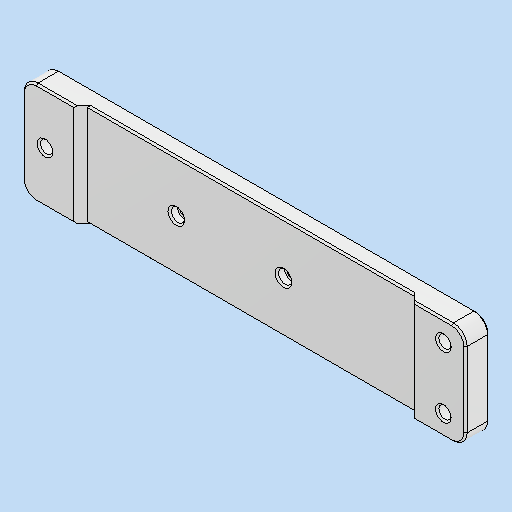
# Autodesk Inventor part: LRS-150-din-bracket
Saved by Autodesk Inventor 2026 (Build 300175050, 175E)
## iProperties
Created: 2025-06-13
Part Number: LRS-150-din-bracket
Material: ABS Plastic
Document SubType Name: Modeling
Designer: kuzmin
Density: 1.06 g/cm^3
Appearance: Smooth - White
Author: kuzmin
Autodesk Inventor part; units mm, degrees
ref_plane "YZ Plane" through (0, 0, 0) normal (1, 0, 0) x (0, 1, 0)
ref_plane "XZ Plane" through (0, 0, 0) normal (0, 1, 0) x (-1, 0, 0)
ref_plane "XY Plane" through (0, 0, 0) normal (0, 0, 1) x (1, 0, 0)
sketch "Sketch1" plane through (0, 0, 0) normal (0, 0, 1) x (1, 0, 0)
  line L0 (-65, 15) -> (65, 15)
  line L1 (65, 15) -> (65, -15)
  line L2 (65, -15) -> (-65, -15)
  line L3 (-65, -15) -> (-65, 15)
  point P0 (0, 0)
  point P1 (0, 15)
  point P2 (65, 0)
  dimension "d0" = 130
  dimension "d1" = 30
  constraints: 8 end point, 2 midpoint, 2 parallel, 1 horizontal, 1 horizontal alignment, 1 perpendicular, 1 vertical alignment
  measures "d0" distance of L0.start L0.end
  measures "d1" distance of L0.end L1.end
extrude "Extrusion1" add sketch "Sketch1" along normal blind 7
sketch "Sketch2" plane through (0, 0, 7) normal (0, 0, 1) x (1, 0, 0)
  line L0 (58.5, 9) -> (58.5, -9) construction
  line L1 (-58.5, 0) -> (58.5, 0) construction
  point P0 (0, 0)
  point P1 (0, 0)
  dimension "d4" = 117
  dimension "d5" = 18
  constraints: 4 coincident, 4 end point, 2 midpoint, 1 horizontal, 1 vertical
  measures "d4" distance of L1.start L1.end
  measures "d5" distance of L0.start L0.end
hole "Hole1" at (-58.5, 0, 7) at (58.5, 9, 7) at (58.5, -9, 7) direction (0, 0, -1) diameter 3.6 end through all
sketch "Sketch3" plane through (0, 0, 7) normal (0, 0, 1) x (1, 0, 0)
  line L0 (65, 15) -> (-65, 15) projected
  line L1 (-65, -15) -> (65, -15) projected
  line L2 (-50, 15) -> (50, 15)
  line L3 (50, 15) -> (50, -15)
  line L4 (50, -15) -> (-50, -15)
  line L5 (-50, -15) -> (-50, 15)
  point P0 (0, 0)
  point P1 (0, -15)
  dimension "d13" = 100
  constraints: 8 end point, 2 parallel, 2 point on line, 1 horizontal, 1 midpoint, 1 perpendicular, 1 vertical alignment
  measures "d13" distance between parallel lines of L3 L5
extrude "Extrusion2" cut sketch "Sketch3" against normal blind 2
sketch "Sketch4" plane through (0, 0, 5) normal (0, 0, 1) x (1, 0, 0)
  line L0 (-21.9201, 0) -> (9.5799, 0) construction
  point P0 (0, 0)
  dimension "d16" = 31.5
  constraints: 2 coincident, 2 end point, 1 horizontal
  measures "d16" distance of L0.start L0.end
hole "Hole2" at (-21.9201, 0, 5) at (9.5799, 0, 5) direction (0, 0, -1) diameter 2.5 end through all counterbore diameter 3.9 counterbore depth 2.3
fillet "Fillet1" radius 4 4 edges at (-65, -15, 3.5) (-65, 15, 3.5) (65, 15, 3.5) (65, -15, 3.5)
chamfer "Chamfer1" distance 2 angle 45 2 edges at (-50, 0, 5) (50, 0, 5)
chamfer "Chamfer2" distance 0.5 angle 45 10 edges at (-21.9201, 1.95, 5) (9.5799, 1.95, 5) (58.5, -7.2, 7) (58.5, 10.8, 7) (-58.5, 1.8, 7) (58.5, -7.2, 0) (-58.5, 1.8, 0) (58.5, 10.8, 0) (-21.9201, 1.25, 0) (9.5799, 1.25, 0)
chamfer "Chamfer3" distance 0.5 angle 45 20 edges at (0, 15, 5) (-55.5, 15, 7) (-63.8284, 13.8284, 7) (-65, 0, 7) (-63.8284, -13.8284, 7) (-55.5, -15, 7) (0, -15, 5) (55.5, 15, 7) (63.8284, 13.8284, 7) (65, 0, 7) (63.8284, -13.8284, 7) (55.5, -15, 7) (0, 15, 0) (-63.8284, 13.8284, 0) (-65, 0, 0) (-63.8284, -13.8284, 0) (0, -15, 0) (63.8284, -13.8284, 0) (65, 0, 0) (63.8284, 13.8284, 0)
body "Solid1"
